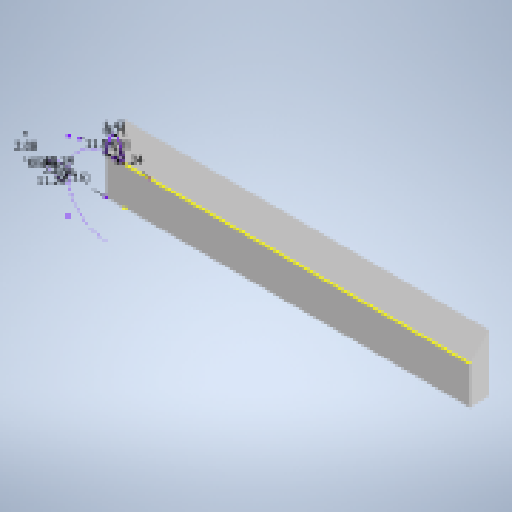
# Autodesk Inventor part: lockPin
Saved by Autodesk Inventor 2023 (Build 270158000, 158)
## iProperties
Created: 2022-11-18
Part Number: lockPin
Material: Generic
Document SubType Name: Modeling
Designer: shrey
Density: 1 g/cm^3
Appearance: Default
Author: shrey
Autodesk Inventor part; units mm, degrees
ref_plane "YZ Plane" through (0, 0, 0) normal (1, 0, 0) x (0, 1, 0)
ref_plane "XZ Plane" through (0, 0, 0) normal (0, 1, 0) x (-1, 0, 0)
ref_plane "XY Plane" through (0, 0, 0) normal (0, 0, 1) x (1, 0, 0)
sketch "Sketch1" plane through (0, 0, 0) normal (1, 0, 0) x (0, 1, 0)
  line L0 (0, 0) -> (15, 0)
  line L1 (15, 0) -> (15, 5)
  line L2 (15, 5) -> (0, 5)
  line L3 (0, 5) -> (0, 0)
  line L4 (10, 5) -> (15, 0)
  dimension "d0" = 15
  dimension "d1" = 5
  dimension "d2" = 5
  constraints: 10 end point, 2 parallel, 1 horizontal, 1 perpendicular, 1 point on line
  measures "d0" distance of L2.end L1.end
  measures "d1" distance of L1.end L0.end
  measures "d2" distance from line of L1 L4.start
extrude "Extrusion1" add sketch "Sketch1" along normal blind 90 and the other way blind 5 contours L3 L2 L4 L0
sketch "Sketch2" plane through (-5, 0, 5) normal (0, 0, 1) x (1, 0, 0)
  arc A0 (0, 10) -> (0, -10) centre (0, 0) ccw construction
  arc A1 (-9.7813, 2.08) -> (-9.7813, -2.08) centre (0, 0) ccw construction
  arc A2 (-15.2728, 0.745) -> (-15.2761, -0.675) centre (0, 0) ccw construction
  arc A3 (-15.2761, -0.675) -> (-9.7813, -2.08) centre (-9.8343, 9.1599) ccw construction
  arc A4 (-9.7813, 2.08) -> (-15.2728, 0.745) centre (-9.9572, -9.1586) ccw construction
  line L0 (0, 10) -> (4.16, 10)
  line L1 (0, 10) -> (95, 10) projected
  line L2 (1.37, 15.291) -> (2.79, 15.291)
  arc A5 (1.37, 15.291) -> (0, 10) centre (11.2397, 9.9126) ccw
  arc A6 (4.16, 10) -> (2.79, 15.291) centre (-7.0797, 9.9126) ccw
  point P0 (5, 0)
  point P1 (2.08, 10)
  dimension "d7" = 4.16
  dimension "d8" = 2.08
  dimension "d9" = 0.745
  dimension "d10" = 1.42
  dimension "d12" = 11.24
  dimension "d13" = 11.24
  dimension "d14" = 5.291
  dimension "d15" = 4.16
  dimension "d16" = 4.16
  dimension "d17" = 1.42
  dimension "d18" = 0.71
  dimension "d19" = 5.291
  dimension "d20" = 11.24
  dimension "d21" = 11.24
  constraints: 16 point on circle, 7 centre point, 4 end point, 1 coincident, 1 horizontal, 1 midpoint, 1 point on line
  measures "d7" distance of A1.start A1.end
  measures "d8" vertical distance of A1.centre A1.start
  measures "d9" vertical distance of A1.centre A2.start
  measures "d10" distance of A2.start A2.end
  measures "d12" radius of A3
  measures "d13" radius of A4
  measures "d14" radial gap between concentric circles of A2 A0
  measures "d15" distance of A1.end A1.start
  measures "d16" distance of L0.start L0.end
  measures "d17" distance of L2.start L2.end
  measures "d18" horizontal distance of L2.end point (2.08, 10)
  measures "d19" distance between parallel lines of L2 L0
  measures "d20" radius of A5
  measures "d21" radius of A6
sketch "Sketch3" plane through (90, 15, 0) normal (0, 0, -1) x (-1, 0, 0)
  arc A0 (0, 1.075) -> (0, -1.075) centre (0, 0) ccw
  arc A1 (-14.714, 2.915) -> (-14.714, -2.915) centre (0, 0) ccw
  arc A2 (-21.0975, 0.975) -> (-21.0975, -0.975) centre (0, 0) ccw
  arc A3 (-21.0975, -0.975) -> (-14.714, -2.915) centre (-14.5146, 9.2134) ccw
  arc A4 (-14.714, 2.915) -> (-21.0975, 0.975) centre (-14.5146, -9.2134) ccw
  arc A5 (0, 1.075) -> (0, -1.075) centre (0, 0) ccw
  arc A6 (-14.714, 2.915) -> (-14.714, -2.915) centre (0, 0) ccw
  arc A7 (-21.0975, 0.975) -> (-21.0975, -0.975) centre (0, 0) ccw
  arc A8 (-21.0975, -0.975) -> (-14.714, -2.915) centre (-14.5146, 9.2134) ccw
  arc A9 (-14.714, 2.915) -> (-21.0975, 0.975) centre (-14.5146, -9.2134) ccw
  line L0 (0, 0) -> (95, 0) projected
  line L1 (95, 0) -> (89.17, 0)
  line L2 (91.11, 6.12) -> (93.06, 6.12)
  arc A10 (91.11, 6.12) -> (89.17, 0) centre (101.2907, -0.4747) ccw
  arc A11 (95, 0) -> (93.06, 6.12) centre (82.8793, -0.4747) ccw
  point P0 (90, -15)
  point P1 (0, -15)
  point P2 (0, -15)
  point P3 (92.085, 0)
  dimension "d22" = 2.915
  dimension "d23" = 5.83
  dimension "d24" = 0.975
  dimension "d25" = 1.95
  dimension "d26" = 21.12
  dimension "d27" = 12.13
  dimension "d28" = 12.13
  dimension "d29" = 2.915
  dimension "d30" = 5.83
  dimension "d31" = 0.975
  dimension "d32" = 1.95
  dimension "d33" = 21.12
  dimension "d34" = 12.13
  dimension "d35" = 12.13
  dimension "d36" = 5.83
  dimension "d37" = 5.83
  dimension "d38" = 1.95
  dimension "d39" = 0.975
  dimension "d40" = 6.12
  dimension "d41" = 6.12
  dimension "d42" = 12.13
  dimension "d43" = 12.13
  constraints: 24 point on circle, 12 centre point, 4 coincident, 4 end point, 1 horizontal, 1 midpoint, 1 point on line
  measures "d22" vertical distance of L0.start A1.end
  measures "d23" distance of A1.end A1.start
  measures "d24" vertical distance of L0.start A2.start
  measures "d25" distance of A2.start A2.end
  measures "d26" radius of A2
  measures "d27" radius of A3
  measures "d28" radius of A4
  measures "d29" vertical distance of A6.centre A6.end
  measures "d30" distance of A6.end A6.start
  measures "d31" vertical distance of A6.centre A7.start
  measures "d32" distance of A7.start A7.end
  measures "d33" radius of A7
  measures "d34" radius of A8
  measures "d35" radius of A9
  measures "d36" distance of A1.start A6.end
  measures "d37" distance of L0.end L1.end
  measures "d38" distance of L2.start L2.end
  measures "d39" horizontal distance of L2.end point (92.085, 0)
  measures "d40" radial gap between concentric circles of A2 A1
  measures "d41" distance between parallel lines of L2 L0
  measures "d42" radius of A10
  measures "d43" radius of A11
loft "Loft1" add profiles "Sketch2", "Sketch3" contours all / A10 L2 A11 L0
pattern_linear "Rectangular Pattern1" count 11 spacing 8.91 along (1, 0, 0) of "Loft1"
body "Solid1"
